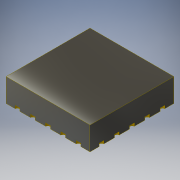
# Autodesk Inventor part: MC_JG1228
Saved by Autodesk Inventor 2016 (Build 200138000, 138)
## iProperties
Created: 2016-08-30
Part Number: MC_JG1228
Material: Generic
Document SubType Name: Modeling
Designer: jfixelle
Density: 1 g/cm^3
Appearance: Silver
Author: jfixelle
Autodesk Inventor part; units mm, degrees
ref_plane "YZ Plane" through (0, 0, 0) normal (1, 0, 0) x (0, 1, 0)
ref_plane "XZ Plane" through (0, 0, 0) normal (0, 1, 0) x (-1, 0, 0)
ref_plane "XY Plane" through (0, 0, 0) normal (0, 0, 1) x (1, 0, 0)
sketch "Sketch1" plane through (0, 0, 0) normal (0, 1, 0) x (-1, 0, 0)
  line L0 (11.555, 11.555) -> (-11.555, 11.555)
  line L1 (-11.555, 11.555) -> (-11.555, -11.555)
  line L2 (-11.555, -11.555) -> (11.555, -11.555)
  line L3 (11.555, -11.555) -> (11.555, 11.555)
  point P0 (0, 0)
  dimension "d0" = 23.11
  dimension "d1" = 23.11
  dimension "d2" = 11.555
  dimension "d3" = 11.555
  constraints: 8 end point, 2 parallel, 1 horizontal, 1 perpendicular
  measures "d0" distance of L2.end L0.start
  measures "d1" distance of L1.end L2.end
  measures "d2" distance from line of point (0, 0) L3
  measures "d3" distance from line of point (0, 0) L2
extrude "Extrusion1" add sketch "Sketch1" along normal blind 6.4
sketch "Sketch2" plane through (0, 0, 0) normal (0, -1, 0) x (1, 0, 0)
  line L0 (11.605, 9.135) -> (10.135, 9.135)
  line L1 (10.135, 9.135) -> (10.135, 7.615)
  line L2 (10.135, 7.615) -> (11.605, 7.615)
  line L3 (11.605, 7.615) -> (11.605, 9.135)
  line L4 (11.555, 11.555) -> (11.555, -11.555) projected
  line L5 (-11.555, 11.555) -> (11.555, 11.555) projected
  circle A0 centre (11.605, 8.375) radius 0.6568
  point P0 (0, 0)
  dimension "d6" = 1.52
  dimension "d7" = 1.47
  dimension "d8" = 0.05
  dimension "d9" = 2.42
  constraints: 8 end point, 2 parallel, 1 centre point, 1 horizontal, 1 midpoint, 1 perpendicular
  measures "d6" distance of L2.end L0.start
  measures "d7" distance of L1.end L2.end
  measures "d8" distance between parallel lines of L4 L3
  measures "d9" distance between parallel lines of L0 L5
extrude "Extrusion2" cut sketch "Sketch2" against normal blind 0.8 contours A0 L3 | L3 A0 L4 | L4 A0
pattern_linear "Rectangular Pattern1" count 5 spacing 4.19 along (0, 0, -1) of "Extrusion2"
pattern_circular "Circular Pattern1" count 4 over 360 about axis through (0, -10, 0) along (0, 1, 0) of "Extrusion2", "Rectangular Pattern1"
body "Solid1"
